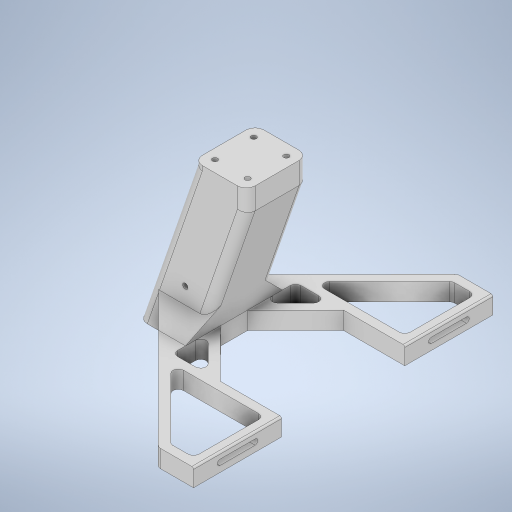
# Autodesk Inventor part: UpperLandingLegMount - BranchBrace+Shortened
Saved by Autodesk Inventor 2023 (Build 270158000, 158)
## iProperties
Created: 2023-01-11
Part Number: UpperLandingLegMount - BranchBrace+Shortened
Material: Generic
Document SubType Name: Modeling
Designer: chase
Density: 1 g/cm^3
Appearance: Default
Author: chase
Autodesk Inventor part; units mm, degrees
ref_plane "YZ Plane" through (0, 0, 0) normal (1, 0, 0) x (0, 1, 0)
ref_plane "XZ Plane" through (0, 0, 0) normal (0, 1, 0) x (-1, 0, 0)
ref_plane "XY Plane" through (0, 0, 0) normal (0, 0, 1) x (1, 0, 0)
sketch "Sketch1" plane through (0, 0, 0) normal (0, 0, 1) x (1, 0, 0)
  circle A0 centre (5.75, 0) radius 1.35 construction
  circle A1 centre (5.75, 0) radius 1.5
  circle A2 centre (24.25, 0) radius 1.55 construction
  circle A3 centre (24.25, 0) radius 1.5
  circle A4 centre (24.25, 22) radius 1.55 construction
  circle A5 centre (24.25, 22) radius 1.5
  circle A6 centre (5.75, 22) radius 1.35 construction
  circle A7 centre (5.75, 22) radius 1.5
  line L0 (5.75, 0) -> (0, 0) construction
  line L1 (0, 35.2322) -> (0, -14.7678) construction
  line L2 (5.75, 22) -> (24.25, 22) construction
  line L3 (24.25, 22) -> (24.25, 0) construction
  line L4 (24.25, 0) -> (5.75, 0) construction
  line L5 (5.75, 0) -> (5.75, 22) construction
  line L6 (0, -6.5) -> (30, -6.5)
  line L7 (30, -6.5) -> (30, 28.5)
  line L8 (30, 28.5) -> (0, 28.5)
  line L9 (0, 28.5) -> (0, -6.5)
  line L10 (30, 28.5) -> (30, 28.5)
  line L11 (30, 11) -> (0, 11) construction
  line L12 (0, 36) -> (5.124, 36)
  line L13 (0, -14) -> (5.124, -14)
  line L14 (0, 28.5) -> (0, 36)
  line L15 (5.124, 36) -> (23.4965, 67.8221)
  line L16 (5.124, -14) -> (23.4965, -45.8221)
  line L17 (16.6, 31.649) -> (16.6, 40.549)
  line L18 (16.6, 40.549) -> (18.8148, 40.549)
  line L19 (16.6, 31.649) -> (18.8148, 31.649)
  circle A8 centre (16.6, 40.549) radius 1.55
  circle A9 centre (16.6, 31.649) radius 1.55
  line L20 (16.6, -9.649) -> (16.6, -18.549)
  line L21 (16.6, -18.549) -> (18.8148, -18.549)
  line L22 (16.6, -9.649) -> (18.8148, -9.649)
  circle A10 centre (16.6, -18.549) radius 1.55
  circle A11 centre (16.6, -9.649) radius 1.55
  line L23 (23.4965, 67.8221) -> (28.6927, 64.8221)
  line L24 (16.6, 40.549) -> (16.6, 31.649) construction
  arc A12 (18.15, 40.549) -> (15.05, 40.549) centre (16.6, 40.549) ccw
  arc A13 (15.05, 31.649) -> (18.15, 31.649) centre (16.6, 31.649) ccw
  line L25 (28.6927, 64.8221) -> (23.9013, 28.5)
  line L26 (23.4965, -45.8221) -> (28.6927, -42.8221)
  line L27 (28.6927, -42.8221) -> (23.9013, -6.5)
  line L28 (0, -6.5) -> (0, -14)
  point P0 (0, 0)
  point P1 (0, 0)
  point P2 (16.6, -6.5)
  point P3 (16.6, -25.1317)
  point P4 (16.6, 36.099)
  dimension "d0" = 3
  dimension "d1" = 3
  dimension "d2" = 3
  dimension "d3" = 3
  dimension "d4" = 30
  dimension "d5" = 35
  dimension "d6" = 6.5
  dimension "d7" = 22
  dimension "d8" = 18.5
  dimension "d9" = 0
  dimension "d10" = 0
  dimension "d11" = 5.75
  dimension "d12" = 0
  dimension "d13" = 0
  dimension "d14" = 0
  dimension "d21" = 50
  dimension "d23" = 120
  dimension "d24" = 16.6
  dimension "d26" = 8.9
  dimension "d27" = 3.1
  dimension "d28" = 3.1
  dimension "d31" = 6
  constraints: 60 end point, 14 centre point, 9 symmetric about line, 7 coincident, 7 parallel, 5 point on line, 4 horizontal, 4 point on circle, 3 midpoint, 3 perpendicular, 2 collinear, 1 concentric, 1 vertical, 2 other
  measures "d0" diameter of A1
  measures "d1" diameter of A3
  measures "d2" diameter of A5
  measures "d3" diameter of A7
  measures "d4" distance of L9.end L7.start
  measures "d5" distance of L7.start L7.end
  measures "d6" distance from line of L6 A3.centre
  measures "d7" distance of L3.start L3.end
  measures "d8" distance of L3.end L5.start
  measures "d9" vertical distance of A3.centre A1.centre
  measures "d10" vertical distance of point (0, 0) A1.centre
  measures "d11" distance from line of L1 A1.centre
  measures "d12" horizontal distance of L5.end A1.centre
  measures "d13" distance from line of L1 point (0, 0)
  measures "d14" distance of L7.end L10.end
  measures "d21" distance between parallel lines of L12 L13
  measures "d23" angle of L12 L15
  measures "d24" distance between parallel lines of L14 L17
  measures "d26" distance between parallel lines of L18 L19
  measures "d27" diameter of A8
  measures "d28" diameter of A9
  measures "d31" distance of L15.end L23.end
extrude "Extrusion: MountFace" add sketch "Sketch1" against normal blind 2 contours L9 L8 L7 L6
draft "FaceDraft1" angle 18.99 pull direction (-1, 0, 0) fixed plane through (0, 16.8333, -0.6667) normal (-1, 0, 0) faces at (12.2007, 14.2552, -2)
ref_plane "Work Plane: Vert" through (0, 11, 0) normal (0, 1, 0) x (1, 0, 0)
ref_plane "Work Plane: Base" through (-37.7144, 11, -158.2304) normal (-0.3254031, 0, -0.9455754) x (-0.9455754, 0, 0.3254031)
ref_plane "Work Plane: Brace" through (0, 0, -88.5) normal (0, 0, 1) x (1, 0, 0)
sketch "Sketch12" plane through (0, 0, -88.5) normal (0, 0, 1) x (1, 0, 0)
  line L0 (67.544, 96) -> (67.544, -74)
  ellipse E0 centre (-37.7144, 11) end of major axis (-37.7144, 22) minor radius 10.4013 (-30.7287, 2.8501) -> (-30.7287, 19.1499) ccw projected
  line L1 (67.544, 96) -> (47.544, 96)
  line L2 (47.544, 96) -> (47.544, -74)
  line L3 (47.544, -74) -> (67.544, -74)
  line L4 (67.544, -74) -> (67.544, 96)
  line L5 (-25.1358, -1.2423) -> (47.544, -74)
  line L6 (-25.1358, 23.2423) -> (47.544, 96)
  line L7 (52.544, -69) -> (62.544, -69)
  line L8 (62.544, -69) -> (62.544, 91)
  line L9 (62.544, 91) -> (52.544, 91)
  line L10 (52.544, 91) -> (52.544, -69)
  line L11 (67.544, -74) -> (67.544, 96)
  line L12 (-22.456, -3.925) -> (-22.456, 25.925)
  point P0 (0, 0)
  point P1 (-27.3131, 11)
  point P2 (23.5, 22)
  point P3 (67.544, -74)
  point P4 (62.544, 11)
  point P5 (67.544, 11)
  dimension "d91" = 170
  dimension "d92" = 85
  dimension "d94" = 44.044
  dimension "d95" = 20
  dimension "d106" = 0
  dimension "d111" = 10
  dimension "d112" = 160
  dimension "d113" = 5
  dimension "d115" = 70
  dimension "d117" = 0
  constraints: 26 end point, 4 parallel, 2 horizontal, 2 midpoint, 2 perpendicular, 2 point on line, 2 vertical, 2 vertical alignment, 4 other
  measures "d91" distance of L0.start L0.end
  measures "d92" vertical distance of point (-27.313, 11) L0.start
  measures "d94" distance from line of L0 point (23.5, 22)
  measures "d95" distance of L3.end L2.end
  measures "d106" distance from line of L0.end L3
  measures "d111" distance of L9.end L8.end
  measures "d112" distance of L8.end L7.end
  measures "d113" distance from line of L11 point (62.544, 11)
  measures "d115" distance between parallel lines of L2 L12
  measures "d117" vertical distance of point (67.544, 11) point (62.544, 11)
extrude "Extrusion: Brace" add sketch "Sketch12" along normal mid plane 10 contours L0 L3 L2 L1 | L2 L5 L12 L6 | L10 L9 L8 L7
sketch "Sketch13" plane through (67.544, -74, -83.5) normal (1, 0, 0) x (0, 0, -1)
  line L0 (0, 0) -> (0, 170) construction
  line L1 (10, 99.925) -> (10, 170) construction
  line L2 (0, 0) -> (10, 170) construction
  line L3 (5, 85) -> (5, 145)
  line L4 (5, 135) -> (5, 155) construction
  line L5 (6.55, 135) -> (6.55, 155)
  line L6 (3.45, 155) -> (3.45, 135)
  arc A0 (3.45, 135) -> (6.55, 135) centre (5, 135) ccw
  arc A1 (6.55, 155) -> (3.45, 155) centre (5, 155) ccw
  line L7 (5, 85) -> (5, 25)
  line L8 (5, 35) -> (5, 15) construction
  line L9 (3.45, 35) -> (3.45, 15)
  line L10 (6.55, 15) -> (6.55, 35)
  arc A2 (6.55, 35) -> (3.45, 35) centre (5, 35) ccw
  arc A3 (3.45, 15) -> (6.55, 15) centre (5, 15) ccw
  point P0 (-83.5, 74)
  point P1 (10, 97.4363)
  dimension "d98" = 60
  dimension "d99" = 10
  dimension "d100" = 3.1
  dimension "d101" = 60
  dimension "d102" = 10
  dimension "d103" = 3.1
  constraints: 22 end point, 8 point on circle, 8 tangent, 4 centre point, 4 vertical, 3 midpoint, 2 parallel
  measures "d98" distance of L3.start L3.end
  measures "d99" distance of L3.end L4.end
  measures "d100" diameter of A1
  measures "d101" distance of L3.start L7.end
  measures "d102" distance of L7.end L8.end
  measures "d103" diameter of A3
extrude "Extrusion: Slots" cut sketch "Sketch13" against normal blind 5
sketch "Sketch17" plane through (0, -6.5, -2) normal (-0.3254031, 0, -0.9455754) x (-0.9455754, 0, 0.3254031)
  line L0 (0, 0) -> (0, 35) projected
  line L1 (-31.7267, 0) -> (0, 0) projected
  line L2 (0, 35) -> (-31.7267, 35)
  line L3 (-31.7267, 35) -> (-31.7267, 0)
  line L4 (-31.7267, 0) -> (0, 0)
  line L5 (0, 0) -> (0, 35)
  point P0 (0.6508, 6.5)
  constraints: 8 end point, 2 parallel, 1 horizontal, 1 perpendicular
extrude "Extrusion: Pillar" add sketch "Sketch17" along normal blind 100
sketch "Sketch15" plane through (0, 0, -83.5) normal (0, 0, 1) x (1, 0, 0)
  line L0 (67.544, -74) -> (47.544, -74) projected
  line L1 (67.544, -74) -> (67.544, 96) projected
  line L2 (47.544, -74) -> (67.544, -74)
  line L3 (67.544, -74) -> (67.544, 96)
  line L4 (-22.456, -3.925) -> (47.544, -74) projected
  line L5 (47.544, -74) -> (-22.456, -3.925)
  line L6 (-30.2977, 11) -> (49.6166, -69)
  line L7 (49.6166, -69) -> (62.544, -69)
  line L8 (62.544, -69) -> (62.544, 101)
  line L9 (-30.2977, 11) -> (49.6166, 91)
  line L10 (47.544, 96) -> (-22.456, 25.925) projected
  line L11 (49.6166, 91) -> (62.544, 91)
  line L12 (67.544, 96) -> (47.544, 96) projected
  line L13 (62.544, -69) -> (57.544, -69)
  line L14 (57.544, -69) -> (57.544, -29)
  line L15 (57.544, -29) -> (62.544, -29)
  line L16 (62.544, -29) -> (62.544, -69)
  line L17 (62.544, 91) -> (57.544, 91)
  line L18 (57.544, 91) -> (57.544, 51)
  line L19 (57.544, 51) -> (62.544, 51)
  line L20 (62.544, 51) -> (62.544, 91)
  line L21 (57.544, -29) -> (9.6595, -29)
  line L22 (4.6648, -24) -> (62.544, -24)
  line L23 (4.6648, 46) -> (62.544, 46)
  line L24 (9.6595, 51) -> (57.544, 51)
  line L25 (-19.8837, 28.5) -> (47.544, 96) projected
  line L26 (47.544, 96) -> (67.544, 96) projected
  line L27 (67.544, 96) -> (67.544, -74) projected
  line L28 (67.544, -74) -> (47.544, -74) projected
  line L29 (47.544, -74) -> (-19.8837, -6.5) projected
  line L30 (5.506, -6.5) -> (-19.8837, -6.5) projected
  line L31 (5.506, 28.5) -> (5.506, -6.5) projected
  line L32 (-19.8837, 28.5) -> (5.506, 28.5) projected
  line L33 (-28.0468, 28.5) -> (-19.8837, 28.5) projected
  line L34 (-28.0468, -6.5) -> (-28.0468, 28.5) projected
  line L35 (-19.8837, -6.5) -> (-28.0468, -6.5) projected
  line L36 (-19.8837, 28.5) -> (5.506, 28.5) projected
  line L37 (62.544, -24) -> (67.544, -24)
  line L38 (62.544, 46) -> (67.544, 46)
  line L39 (5.506, 28.5) -> (5.506, -6.5) projected
  line L40 (12.0647, 6.9754) -> (12.0647, 15.0246)
  line L41 (2.0647, -6.5) -> (2.0647, 28.5) projected
  line L42 (5.506, 5.1337) -> (5.506, -24)
  line L43 (5.506, 16.8663) -> (5.506, 46)
  line L44 (25.8667, -24) -> (5.506, -3.6175)
  line L45 (5.506, 25.6175) -> (25.8667, 46)
  line L46 (32.934, -24) -> (5.506, 3.4573)
  line L47 (5.506, 18.5427) -> (32.934, 46)
  point P0 (0, 0)
  point P1 (33.6017, 51)
  point P2 (62.544, 51)
  point P3 (62.544, -29)
  point P4 (67.544, 46)
  point P5 (57.544, 91)
  point P6 (15.6863, -13.8088)
  point P7 (15.6863, 35.8088)
  point P8 (5.506, 3.4573)
  point P9 (5.506, -3.6175)
  dimension "d119" = 5
  dimension "d120" = 5
  dimension "d121" = 5
  dimension "d122" = 5
  dimension "d123" = 5
  dimension "d124" = 5
  dimension "d125" = 40
  dimension "d126" = 40
  dimension "d127" = 5
  dimension "d128" = 5
  dimension "d157" = 15
  dimension "d158" = 15
  dimension "d159" = 5
  dimension "d160" = 5
  constraints: 58 end point, 20 point on line, 12 parallel, 8 horizontal, 5 midpoint, 5 perpendicular, 2 collinear, 2 other
  measures "d119" distance between parallel lines of L4 L6
  measures "d120" distance between parallel lines of L2 L7
  measures "d121" distance between parallel lines of L1 L8
  measures "d122" distance between parallel lines of L10 L9
  measures "d124" distance of L14.end L15.end
  measures "d125" distance of L13.end L14.end
  measures "d126" distance of L18.end L17.end
  measures "d127" distance between parallel lines of L22 L21
  measures "d128" distance from line of point (33.602, 51) L23
  measures "d157" distance from line of point (15.686, -13.809) L6
  measures "d158" distance from line of L9 point (15.686, 35.809)
  measures "d159" distance between parallel lines of L44 L46
  measures "d160" distance between parallel lines of L45 L47
extrude "Extrusion: Lightening" cut sketch "Sketch15" against normal up to surface (10 mm away) contours L37 L8 L38 L1 | L22 L46 L31 L47 L23 L8 | L8 L7 L14 L15 | L19 L18 L11 L8 | L14 L7 L6 L21 | L22 L42 L31 L44 | L24 L9 L11 L18 | L45 L31 L43 L23
sketch "Sketch16" plane through (0, 0, -93.5) normal (0, 0, -1) x (-1, 0, 0)
  line L0 (65.3576, 48.2147) -> (-32.3626, 48.2147)
  line L1 (-32.3626, 48.2147) -> (-32.3626, -28.742)
  line L2 (-32.3626, -28.742) -> (65.3576, -28.742)
  line L3 (65.3576, -28.742) -> (65.3576, 48.2147)
  point P0 (0, 0)
  constraints: 8 end point, 2 parallel, 1 horizontal, 1 perpendicular
extrude "Extrusion: RemoveBot" cut sketch "Sketch16" along normal through all
sketch "Sketch18" plane through (-37.7144, 11, -158.2304) normal (-0.3254031, 0, -0.9455754) x (-0.9455754, 0, 0.3254031)
  circle A0 centre (0, 0) radius 8.125
  point P0 (15.8269, -11)
  dimension "d137" = 16.25
  constraints: 1 centre point
  measures "d137" diameter of A0
extrude "Extrusion: Tube" cut sketch "Sketch18" against normal blind 110
sketch "Sketch19" plane through (0, -6.5, 0) normal (0, -1, 0) x (1, 0, 0)
  line L0 (0, -2) -> (-31.4881, -93.5) construction
  line L1 (-19.6025, -58.9622) -> (10.3975, -69.2862) construction
  line L2 (30, -12.324) -> (5.506, -83.5) construction
  circle A0 centre (-4.6025, -64.1242) radius 1.5
  point P0 (0, 0)
  dimension "d140" = 3
  constraints: 2 end point, 2 point on line, 1 centre point, 1 midpoint
  measures "d140" diameter of A0
extrude "Extrusion: Pin" cut sketch "Sketch19" against normal up to surface (35 mm away)
chamfer "Chamfer: PillarSupport" distance 10 angle 45 2 edges at (-7.1888, -6.5, -83.5) (-7.1888, 28.5, -83.5)
fillet "Fillet: Pillar" radius 5 8 edges at (-15.7441, 28.5, -47.75) (-15.7441, -6.5, -47.75) (0, 28.5, -1) (0, -6.5, -1) (19.4737, 28.5, -42.912) (19.4737, -6.5, -42.912) (30, -6.5, -6.162) (30, 28.5, -6.162)
fillet "Fillet: SlotLip" radius 1 2 edges at (67.544, 71, -83.5) (67.544, -49, -83.5)
fillet "Fillet: 3mmCorners" radius 3 16 edges at (9.6595, -29, -88.5) (9.6595, 51, -88.5) (5.506, 46, -88.5) (5.506, -24, -88.5) (49.6166, -69, -88.5) (49.6166, 91, -88.5) (47.544, 96, -88.5) (47.544, -74, -88.5) (25.8667, -24, -88.5) (5.506, -3.6175, -88.5) (5.506, 25.6175, -88.5) (25.8667, 46, -88.5) (62.544, -29, -88.5) (62.544, -69, -88.5) (62.544, 51, -88.5) (62.544, 91, -88.5)
equation "\"d6\" = -0.5 * d7 + 0.5 * d5"
equation "\"d11\" = -0.5 * d8 + 0.5 * d4"
equation "\"d92\" = 0.5 * d91"
body "Solid1"
